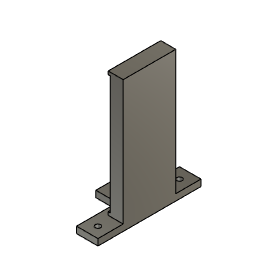
bus_bar_holder (Autodesk Fusion 360 design; units mm, degrees)
Autodesk Fusion 360 part; units mm, degrees
sketch "Sketch8" plane through (0, 0, 0) normal (0, 0, 1) x (1, 0, 0)
  line L0 (0, 0) -> (20, 0)
  line L1 (20, 0) -> (20, 96)
  line L2 (20, 96) -> (0, 96)
  line L3 (0, 96) -> (0, 0)
  line L4 (0, 48) -> (-20, 48) construction
  line L5 (-20, 48) -> (-20, 58) construction
  line L6 (-20, 58) -> (0, 58)
  line L7 (0, 58) -> (0, 38)
  line L8 (0, 38) -> (-20, 38)
  line L9 (-20, 38) -> (-20, 58)
  line L10 (-20, 58) -> (0, 38) construction
  circle A0 centre (-10, 48) radius 2.5
  line L11 (0, 96) -> (20, 76) construction
  line L12 (0, 96) -> (28.2843, 96) construction
  circle A1 centre (10, 86) radius 2.5
  circle A2 centre (10, 10) radius 2.5
  dimension "d44" = 20
  dimension "d45" = 96
  dimension "d46" = 20
  dimension "d47" = 10
  dimension "d48" = 20
  dimension "d49" = 20
  dimension "d50" = 5
  dimension "d51" = 45
  dimension "d52" = 5
  constraint horizontal L0
  constraint vertical L1
  constraint horizontal L2
  constraint vertical L3
  constraint coincident L0.start L3.end
  constraint midpoint L3 L4.start
  constraint perpendicular L3 L4
  constraint perpendicular L4 L5
  constraint horizontal L6
  constraint vertical L7
  constraint horizontal L8
  constraint vertical L9
  constraint midpoint L4 A0.centre
  constraint horizontal L12
  constraint coincident L1 L11.end
  constraint midpoint L11 A1.centre
  constraint symmetric L4 A1 A2
  measures "d44" distance of L0.start L0.end
  measures "d45" distance of L0.start L2.end
  measures "d46" distance of L4.start L4.end
  measures "d47" distance of L4.end L5.end
  measures "d48" distance of L5.end L6.end
  measures "d49" distance of L5.end L8.end
  measures "d50" diameter of A0
  measures "d51" angle of L11 L12
  measures "d52" diameter of A1
extrude "Extrude10" add sketch "Sketch8" along normal blind 6
sketch "Sketch9" plane through (0, 0, 6) normal (0, 0, 1) x (-1, 0, 0)
  circle A0 centre (10, -48) radius 2.5
  circle A1 centre (-10, -10) radius 2.5
  circle A2 centre (-10, -86) radius 2.5
  line L0 (0, -38) -> (0, 0)
  line L1 (0, 0) -> (-20, 0)
  line L2 (-20, 0) -> (-20, -96)
  line L3 (-20, -96) -> (0, -96)
  line L4 (0, -96) -> (0, -58)
  line L5 (0, -58) -> (20, -58)
  line L6 (20, -58) -> (20, -38)
  line L7 (20, -38) -> (0, -38)
  line L8 (-20, -48) -> (20, -48) construction
  line L9 (-20, -48) -> (-20, -52) construction
  line L10 (-20, -52) -> (-6, -52)
  line L11 (-6, -52) -> (-6, -72.5)
  line L12 (-6, -72.5) -> (-20, -72.5)
  line L13 (-20, -72.5) -> (-20, -52)
  line L14 (-20, -44) -> (-6, -44)
  line L15 (-6, -44) -> (-6, -23.5)
  line L16 (-6, -23.5) -> (-20, -23.5)
  dimension "d55" = 4
  dimension "d57" = 14
  dimension "d58" = 20.5
  constraint midpoint L2 L8.start
  constraint midpoint L6 L8.end
  constraint perpendicular L8 L9
  constraint horizontal L10
  constraint vertical L11
  constraint horizontal L12
  constraint vertical L13
  constraint symmetric L8 L9.end L14.start
  constraint symmetric L8 L10.end L14.end
  constraint symmetric L8 L11.end L15.end
  constraint symmetric L8 L12.end L16.end
  measures "d55" distance of L8.start L9.end
  measures "d57" distance of L9.end L10.end
  measures "d58" distance of L9.end L12.end
extrude "Extrude11" add sketch "Sketch9" along normal blind 116.5 contours L2 L14 L15 L16 | L2 L10 L11 L12 L13
sketch "Sketch10" plane through (0, 0, 122.5) normal (0, 0, 1) x (-1, 0, 0)
  line L0 (-6, -23.5) -> (-20, -23.5)
  line L1 (-20, -23.5) -> (-20, -44)
  line L2 (-20, -44) -> (-6, -44)
  line L3 (-6, -44) -> (-6, -23.5)
  line L4 (-20, -72.5) -> (-6, -72.5)
  line L5 (-6, -72.5) -> (-6, -52)
  line L6 (-6, -52) -> (-20, -52)
  line L7 (-20, -52) -> (-20, -72.5)
  line L8 (-6, -72.5) -> (-20, -72.5)
  line L9 (-20, -72.5) -> (-20, -23.5)
  line L10 (-20, -23.5) -> (-6, -23.5)
  line L11 (-6, -23.5) -> (-6, -72.5)
  constraint horizontal L8
  constraint vertical L9
  constraint horizontal L10
  constraint vertical L11
  constraint coincident L0.end L1.start
  constraint coincident L4.end L5.start
extrude "Extrude12" add sketch "Sketch10" against normal blind 3
sketch "Sketch11" plane through (20, 0, 0) normal (1, 0, 0) x (0, 1, 0)
  line L0 (52, 119.5) -> (52, 6)
  line L1 (52, 6) -> (44, 6)
  line L2 (44, 6) -> (44, 119.5)
  line L3 (72.5, 122.5) -> (23.5, 122.5)
  line L4 (72.5, 6) -> (72.5, 122.5)
  line L5 (44, 119.5) -> (52, 119.5)
  line L6 (23.5, 122.5) -> (23.5, 6)
  line L7 (23.5, 6) -> (0, 6)
  line L8 (0, 6) -> (0, 0)
  line L9 (0, 0) -> (96, 0)
  line L10 (96, 0) -> (96, 6)
  line L11 (96, 6) -> (72.5, 6)
  line L12 (23.5, 6) -> (44, 6) construction
  line L13 (48, 119.5) -> (48, 6) construction
  line L14 (26.5, 119.5) -> (41, 119.5)
  line L15 (41, 119.5) -> (41, 9)
  line L16 (41, 9) -> (26.5, 9)
  line L17 (26.5, 9) -> (26.5, 119.5)
  line L18 (55, 119.5) -> (55, 9)
  line L19 (69.5, 119.5) -> (55, 119.5)
  line L20 (69.5, 9) -> (69.5, 119.5)
  line L21 (55, 9) -> (69.5, 9)
  dimension "d64" = 3
  dimension "d65" = 3
  dimension "d67" = 3
  dimension "d68" = 3
  constraint coincident L6.end L7.start
  constraint coincident L1.end L2.start
  constraint midpoint L5 L13.start
  constraint midpoint L1 L13.end
  constraint horizontal L14
  constraint vertical L15
  constraint horizontal L16
  constraint vertical L17
  constraint symmetric L13 L14.start L19.start
  constraint symmetric L13 L14.end L18.start
  constraint symmetric L13 L15.end L18.end
  constraint symmetric L13 L16.end L20.start
  measures "d64" distance of L12 L16
  measures "d65" distance of L6 L17
  measures "d67" distance of L3 L14
  measures "d68" distance of L2 L15
sketch "Sketch14" plane through (6, 0, 0) normal (-1, 0, 0) x (0, -1, 0)
  line L0 (-72.5, 122.5) -> (-72.5, 6)
  line L1 (-72.5, 6) -> (-52, 6)
  line L2 (-52, 6) -> (-52, 119.5)
  line L3 (-52, 119.5) -> (-44, 119.5)
  line L4 (-44, 119.5) -> (-44, 6)
  line L5 (-44, 6) -> (-23.5, 6)
  line L6 (-23.5, 6) -> (-23.5, 122.5)
  line L7 (-23.5, 122.5) -> (-72.5, 122.5)
  line L8 (-69.5, 9) -> (-69.5, 119.5)
  line L9 (-55, 9) -> (-69.5, 9)
  line L10 (-55, 119.5) -> (-55, 9)
  line L11 (-69.5, 119.5) -> (-55, 119.5)
  line L12 (-26.5, 119.5) -> (-41, 119.5)
  line L13 (-41, 119.5) -> (-41, 9)
  line L14 (-26.5, 9) -> (-26.5, 119.5)
  line L15 (-41, 9) -> (-26.5, 9)
extrude "Extrude13" cut sketch "Sketch14" against normal blind 11 contours L8 L9 L10 L11 | L12 L13 L14 L15
extrude "Extrude14" add 1 faces at (10.6667, 46.6667, 119.5) along direction (0, 0, -1) up to surface (113.5 mm away)
sketch "Sketch15" plane through (17, 0, 0) normal (-1, 0, 0) x (0, -1, 0)
  line L0 (-69.5, 119.5) -> (-69.5, 9)
  line L1 (-69.5, 9) -> (-55, 9)
  line L2 (-55, 9) -> (-55, 119.5)
  line L3 (-55, 119.5) -> (-69.5, 119.5)
  line L4 (-56, 118.5) -> (-68.5, 118.5)
  line L5 (-68.5, 118.5) -> (-68.5, 10)
  line L6 (-68.5, 10) -> (-56, 10)
  line L7 (-56, 10) -> (-56, 118.5)
extrude "Extrude15" add sketch "Sketch15" along normal blind 8
sketch "Sketch16" plane through (17, 0, 0) normal (-1, 0, 0) x (0, -1, 0)
  line L0 (-41, 9) -> (-26.5, 9)
  line L1 (-26.5, 9) -> (-26.5, 119.5)
  line L2 (-26.5, 119.5) -> (-41, 119.5)
  line L3 (-41, 119.5) -> (-41, 9)
  line L4 (-27.5, 118.5) -> (-40, 118.5)
  line L5 (-40, 118.5) -> (-40, 10)
  line L6 (-40, 10) -> (-27.5, 10)
  line L7 (-27.5, 10) -> (-27.5, 118.5)
extrude "Extrude16" add sketch "Sketch16" along normal blind 8
sketch "Sketch17" plane through (6, 0, 0) normal (-1, 0, 0) x (0, -1, 0)
  line L0 (-55, 9) -> (-69.5, 9)
  line L1 (-69.5, 9) -> (-69.5, 119.5)
  line L2 (-69.5, 119.5) -> (-55, 119.5)
  line L3 (-55, 119.5) -> (-55, 9)
  line L4 (-26.5, 119.5) -> (-26.5, 9)
  line L5 (-26.5, 9) -> (-41, 9)
  line L6 (-41, 9) -> (-41, 119.5)
  line L7 (-41, 119.5) -> (-26.5, 119.5)
  line L8 (-72.5, 6) -> (-23.5, 6)
  line L9 (-23.5, 6) -> (-23.5, 122.5)
  line L10 (-23.5, 122.5) -> (-72.5, 122.5)
  line L11 (-72.5, 122.5) -> (-72.5, 6)
  line L12 (-69.5, 9) -> (-72.5, 9)
  line L13 (-26.5, 9) -> (-23.5, 9)
  line L14 (-26.5, 119.5) -> (-23.5, 119.5)
  line L15 (-69.5, 119.5) -> (-72.5, 119.5)
  constraint coincident L0.end L1.start
  constraint coincident L11 L12.end
  constraint perpendicular L11 L12
  constraint coincident L4.end L5.start
  constraint coincident L9 L13.end
  constraint perpendicular L9 L13
  constraint coincident L4.start L7.end
  constraint coincident L9 L14.end
  constraint perpendicular L9 L14
  constraint coincident L1.end L2.start
  constraint coincident L11 L15.end
  constraint perpendicular L11 L15
extrude "Extrude17" cut sketch "Sketch17" against normal blind 2 contours L1 L11 L12 L15 | L4 L9 L13 L14
equation "thickness = 6 mm"
equation "bar_width = 14 mm"
equation "bar_length = 110 mm"
equation "bar_under_depth = 8 mm"
equation "bar_thickness = 3 mm"
equation "bar_shelf_width = 1 mm"
equation "space_between_bars = 8 mm"
equation "frame_width = 96 mm"
equation "extrusion_width = 20 mm"
equation "mounting_hole_size = 5 mm"
equation "d44 = extrusion_width"
equation "d45 = frame_width"
equation "d46 = extrusion_width"
equation "d47 = extrusion_width / 2"
equation "d48 = extrusion_width"
equation "d49 = extrusion_width"
equation "d50 = mounting_hole_size"
equation "d52 = mounting_hole_size"
equation "d53 = thickness"
equation "d55 = space_between_bars / 2"
equation "small_thickness = 3 mm"
equation "d57 = bar_thickness + bar_under_depth + small_thickness"
equation "d58 = bar_width + small_thickness * 2 + tolerance * 2"
equation "tolerance = 0.25 mm"
equation "d60 = bar_length + small_thickness * 2 + tolerance * 2"
equation "d62 = -small_thickness"
equation "d64 = small_thickness"
equation "d65 = small_thickness"
equation "d67 = small_thickness"
equation "d68 = small_thickness"
equation "d69 = -bar_thickness - bar_under_depth"
equation "d74 = bar_under_depth"
equation "d77 = bar_under_depth"
equation "d79 = -bar_shelf_width"
equation "d80 = -bar_shelf_width"
equation "wire_cutout_depth = 2 mm"
equation "d82 = -wire_cutout_depth"
